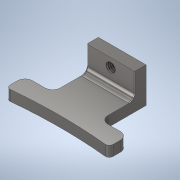
# Autodesk Inventor part: Chip Kick Vorne
Saved by Autodesk Inventor 2020 (Build 240168000, 168)
## iProperties
Part Number: Chip Kick Vorne
Material: Steel, Carbon
Document SubType Name: Modeling
Designer: rYan
Mass: 21.0861 g
Surface Area: 38.1171 cm^2
Volume: 7.80968 cm^3
Density: 7.85 g/cm^3
Appearance: Semi-Polished
Author: rYan
Autodesk Inventor part; units mm, degrees
ref_plane "YZ Plane" through (0, 0, 0) normal (1, 0, 0) x (0, 1, 0)
ref_plane "XZ Plane" through (0, 0, 0) normal (0, 1, 0) x (-1, 0, 0)
ref_plane "XY Plane" through (0, 0, 0) normal (0, 0, 1) x (1, 0, 0)
sketch "Skizze1" plane through (0, 0, 0) normal (1, 0, 0) x (0, 1, 0)
  line L0 (0, 18.5) -> (-6, 18.5)
  line L1 (-6, 18.5) -> (-6, 5.5)
  line L2 (-24, 0) -> (0, 0)
  line L3 (0, 0) -> (0, 18.5)
  line L4 (-24, 0) -> (-24, 5.5)
  line L5 (-24, 5.5) -> (-6, 5.5)
  dimension "d0" = 18.5
  dimension "d1" = 6
  dimension "d2" = 5.5
  dimension "d3" = 24
  constraints: 12 end point, 2 horizontal, 2 parallel, 1 coincident, 1 perpendicular, 1 vertical
  measures "d0" distance of L2.end L0.start
  measures "d1" distance of L0.start L0.end
  measures "d2" distance of L2.start L4.end
  measures "d3" distance of L2.start L2.end
extrude "Extrusion1" add sketch "Skizze1" along normal mid plane 25
sketch "Skizze2" plane through (-12.5, 0, 18.5) normal (0, 1, 0) x (1, 0, 0)
  line L0 (25, 18.5) -> (25, 0) projected
  line L1 (25, 18.5) -> (0, 18.5) projected
  line L2 (0, 0) -> (0, 18.5) projected
  line L3 (0, 0) -> (25, 0) construction
  line L4 (12.5, 0) -> (12.5, 18.5) construction
  line L5 (0, 0) -> (25, 0) projected
  point P0 (12.5, 4.5)
  constraints: 2 end point, 1 midpoint, 1 point on line, 1 vertical
hole "Bohrung1" at (0, 0, 14) direction (0, -1, 0) diameter 4.917 end through all thread size "M6x1" class "6H" standard "ANSI Metric M Profile"
chamfer "Fase1" [suppressed]
fillet "Rundung1" radius 0.5 2 edges at (12.5, -6, 12) (-12.5, -6, 12)
fillet "Rundung2" [suppressed]
sketch "Skizze5" plane through (-12.5, 0, 18.5) normal (0, 1, 0) x (1, 0, 0)
  line L0 (25, 18.5) -> (0, 18.5) projected
  line L1 (0, 0) -> (0, 18.5) projected
  line L2 (25, 18.5) -> (0, 18.5)
  line L3 (0, 18.5) -> (0, 13)
  line L4 (0, 13) -> (25, 13)
  line L5 (25, 13) -> (25, 18.5)
  line L6 (25, 13) -> (25, 18.5) projected
  line L7 (0, 18.5) -> (0, 13) projected
  line L8 (0, 18.5) -> (25, 18.5) projected
  line L9 (0, 13) -> (25, 13) projected
  point P0 (12.5, 18.5)
  point P1 (1, 16.5)
  point P2 (24, 16.5)
  constraints: 8 end point, 2 parallel, 1 horizontal, 1 perpendicular, 1 point on line, 1 other
sketch "Sketch7" plane through (-12.5, -8, 5.5) normal (0, 0, 1) x (1, 0, 0)
  line L0 (25, 8) -> (0, 8) projected
  line L1 (-14.5, -26) -> (39.5, -26) construction
  line L2 (39.5, -26) -> (39.5, -16)
  line L3 (39.5, -16) -> (-14.5, -16)
  line L4 (-14.5, -16) -> (-14.5, -26)
  line L5 (10.0415, 8) -> (14.9585, 8) construction
  line L6 (12.5, 8) -> (12.5, -16) construction
  arc A0 (39.5, -26) -> (-14.5, -26) centre (12.5, -274.5377) ccw
  dimension "d44" = 54
  dimension "d45" = 10
  dimension "d46" = 24
  dimension "d47" = 250
  constraints: 10 end point, 2 midpoint, 2 parallel, 2 point on circle, 1 centre point, 1 horizontal, 1 perpendicular, 1 vertical
  measures "d44" distance of L3.end L2.end
  measures "d45" distance of L2.end L1.end
  measures "d46" distance of L6.end L6.start
  measures "d47" radius of A0
extrude "Extrusion2" add sketch "Sketch7" against normal up to surface (5.5 mm away) from surface at 0
fillet "Fillet3" radius 2 2 edges at (27, -34, 2.75) (-27, -34, 2.75)
fillet "Fillet3" radius 4 4 edges at (12.5, -24, 2.75) (-12.5, -24, 2.75) (27, -24, 2.75) (-27, -24, 2.75)
fillet "Fillet4" radius 3 1 edges at (0, -6, 5.5)
equation "\"d46\" = d3"
